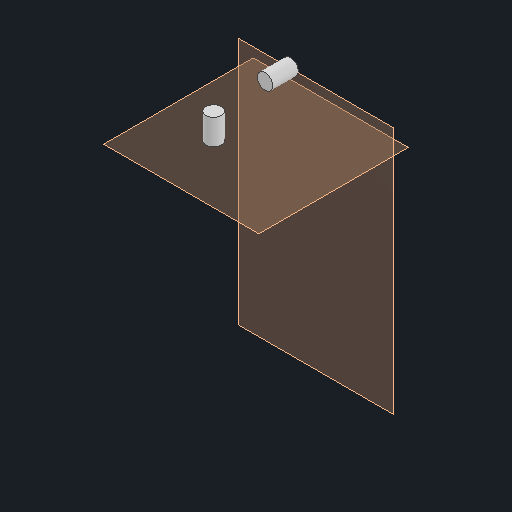
# Autodesk Inventor part: BaseEjeConicos
Saved by Autodesk Inventor 2026.3 (Build 303398000, 398)
## iProperties
Created: 2026-04-17
Part Number: BaseEjeConicos
Material: Genérico
Document SubType Name: Modeling
Designer: Jose Carlos
Density: 1 g/cm^3
Appearance: Valor por defecto
Author: Jose Carlos
Autodesk Inventor part; units mm, degrees
ref_plane "YZ Plane" through (0, 0, 0) normal (1, 0, 0) x (0, 1, 0)
ref_plane "XZ Plane" through (0, 0, 0) normal (0, 1, 0) x (-1, 0, 0)
ref_plane "XY Plane" through (0, 0, 0) normal (0, 0, 1) x (1, 0, 0)
ref_plane "Plano de trabajo1" through (0, 0, 0) normal (0, 0, 1) x (1, 0, 0)
sketch "Boceto1" plane through (0, 0, 0) normal (0, 0, 1) x (1, 0, 0)
  line L0 (-15.5, 39) -> (15.5, 39) construction
  line L1 (0, 35.4) -> (0, 39.6) construction
  circle A0 centre (-10, 49) radius 3
  line L2 (-12.6, 39) -> (-7.4, 39) construction
  point P0 (0, 0)
  point P1 (-10, 39)
  dimension "d0" = 6
  dimension "d1" = 10
  dimension "d7" = 0
  constraints: 2 end point, 1 centre point, 1 midpoint, 1 vertical, 2 other
  measures "d0" diameter of A0
  measures "d1" distance from line of L0 A0.centre
  measures "d7" horizontal distance of point (-10, 39) A0.centre
extrude "Extrusión1" add sketch "Boceto1" along normal blind 10
ref_plane "Plano de trabajo2" through (0, 39, 25) normal (0, 1, 0) x (-1, 0, 0)
sketch "Boceto2" plane through (0, 39, 25) normal (0, 1, 0) x (-1, 0, 0)
  circle A0 centre (10, 5) radius 2.6 construction
  circle A1 centre (10, 5) radius 3
  point P0 (0, -25)
  dimension "d4" = 6
  constraints: 1 centre point, 1 coincident
  measures "d4" diameter of A1
extrude "Extrusión2" add sketch "Boceto2" along normal blind 10
